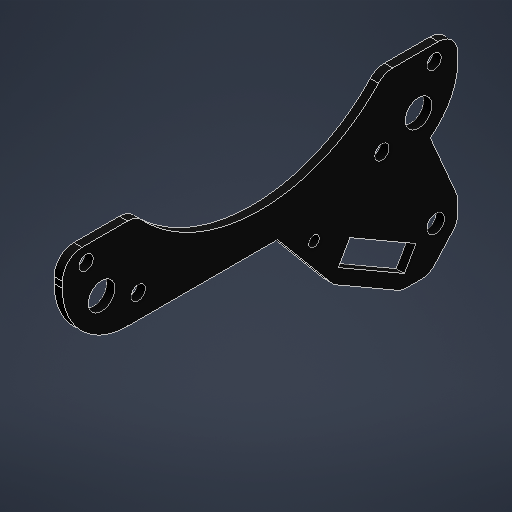
# Autodesk Inventor part: output_support
Saved by Autodesk Inventor 2026.1 (Build 301233000, 233)
## iProperties
Created: 2026-05-06
Part Number: output_support
Material: Generic
Document SubType Name: Modeling
Designer: aaron
Density: 1 g/cm^3
Appearance: Default
Author: aaron
Autodesk Inventor part; units mm, degrees
ref_plane "YZ Plane" through (0, 0, 0) normal (1, 0, 0) x (0, 1, 0)
ref_plane "XZ Plane" through (0, 0, 0) normal (0, 1, 0) x (-1, 0, 0)
sketch "Sketch1" plane through (0, 0, 0) normal (1, 0, 0) x (0, 1, 0)
  line L0 (14.231, -0.0045) -> (14.2475, -121.0044)
  circle A0 centre (46.8483, -60.5) radius 44 projected
  arc A1 (-10.6283, -58.8604) -> (-0.114, -93.6782) centre (46.8483, -60.5) ccw projected
  line L1 (-0.114, -93.6782) -> (2.9975, -94.9709) projected
  arc A2 (2.9975, -94.9709) -> (7.0992, -99.6298) centre (46.8483, -60.5) ccw projected
  line L2 (7.0992, -99.6298) -> (13.2859, -93.5395) projected
  arc A3 (-0.2275, -59.1156) -> (13.2859, -93.5395) centre (46.8483, -60.5) ccw projected
  line L3 (-0.2275, -59.1156) -> (-8.9052, -58.8604) projected
  line L4 (-8.9052, -58.8604) -> (-10.6283, -58.8604) projected
  circle A4 centre (84.1308, -7.2551) radius 2.15 projected
  circle A5 centre (95.3483, -109) radius 2.65 projected
  circle A6 centre (100.0932, -97.7825) radius 2.15 projected
  circle A7 centre (-6.3966, -23.2175) radius 2.15 projected
  circle A8 centre (-6.3966, -97.7825) radius 2.15 projected
  circle A9 centre (-1.6517, -12) radius 2.65 projected
  circle A10 centre (95.3483, -12) radius 2.65 projected
  circle A11 centre (9.5658, -113.7449) radius 2.15 projected
  circle A12 centre (9.5658, -7.2551) radius 2.15 projected
  circle A13 centre (84.1308, -113.7449) radius 2.15 projected
  circle A14 centre (100.0932, -23.2175) radius 2.15 projected
  circle A15 centre (-1.6517, -109) radius 2.65 projected
  line L5 (-7.7476, -49.0794) -> (0.7499, -50.8569) projected
  arc A16 (12.1591, -28.6456) -> (0.7499, -50.8569) centre (46.8483, -60.5) ccw projected
  line L6 (12.1591, -28.6456) -> (5.7646, -22.7737) projected
  arc A17 (5.7646, -22.7737) -> (-7.7476, -49.0794) centre (46.8483, -60.5) ccw projected
  line L7 (83.7453, -102.33) -> (78.0025, -95.8194) projected
  arc A18 (66.2911, -103.3955) -> (78.0025, -95.8194) centre (46.8483, -60.5) ccw projected
  line L8 (66.2911, -103.3955) -> (69.8751, -111.3026) projected
  arc A19 (69.8751, -111.3026) -> (83.7453, -102.33) centre (46.8483, -60.5) ccw projected
  line L9 (85.3896, -20.1799) -> (79.3909, -26.4555) projected
  arc A20 (89.1056, -39.7066) -> (79.3909, -26.4555) centre (46.8483, -60.5) ccw projected
  line L10 (89.1056, -39.7066) -> (96.8951, -35.8737) projected
  arc A21 (96.8951, -35.8737) -> (85.3896, -20.1799) centre (46.8483, -60.5) ccw projected
  line L11 (58.0786, -115.1353) -> (56.3307, -106.6317) projected
  arc A22 (42.4628, -107.3915) -> (56.3307, -106.6317) centre (46.8483, -60.5) ccw projected
  line L12 (42.4628, -107.3915) -> (41.6544, -116.0352) projected
  arc A23 (41.6544, -116.0352) -> (58.0786, -115.1353) centre (46.8483, -60.5) ccw projected
  line L13 (11.1274, -17.6613) -> (16.6872, -24.3288) projected
  arc A24 (31.0571, -16.1301) -> (16.6872, -24.3288) centre (46.8483, -60.5) ccw projected
  line L14 (31.0571, -16.1301) -> (28.1463, -7.9512) projected
  arc A25 (28.1463, -7.9512) -> (11.1274, -17.6613) centre (46.8483, -60.5) ccw projected
  line L15 (101.6271, -71.0083) -> (93.1011, -69.3728) projected
  arc A26 (82.2782, -91.5285) -> (93.1011, -69.3728) centre (46.8483, -60.5) ccw projected
  line L16 (82.2782, -91.5285) -> (88.8092, -97.2481) projected
  arc A27 (88.8092, -97.2481) -> (101.6271, -71.0083) centre (46.8483, -60.5) ccw projected
  line L17 (100.5451, -45.4072) -> (92.1875, -47.7563) projected
  arc A28 (93.8596, -63.3257) -> (92.1875, -47.7563) centre (46.8483, -60.5) ccw projected
  line L18 (93.8596, -63.3257) -> (102.5254, -63.8466) projected
  arc A29 (102.5254, -63.8466) -> (100.5451, -45.4072) centre (46.8483, -60.5) ccw projected
  line L19 (38.2646, -115.6131) -> (39.6006, -107.0351) projected
  arc A30 (20.5997, -99.6032) -> (39.6006, -107.0351) centre (46.8483, -60.5) ccw projected
  line L20 (20.5997, -99.6032) -> (15.7612, -106.8113) projected
  arc A31 (15.7612, -106.8113) -> (38.2646, -115.6131) centre (46.8483, -60.5) ccw projected
  line L21 (38.8508, -5.2987) -> (40.0955, -13.8905) projected
  arc A32 (56.4914, -14.4016) -> (40.0955, -13.8905) centre (46.8483, -60.5) ccw projected
  line L22 (56.4914, -14.4016) -> (58.2689, -5.9041) projected
  arc A33 (58.2689, -5.9041) -> (38.8508, -5.2987) centre (46.8483, -60.5) ccw projected
  arc A34 (6.34, -0.0055) -> (-13.6572, -20.0083) centre (6.3428, -20.0055) ccw projected
  line L23 (6.34, -0.0055) -> (87.34, 0.0055) projected
  arc A35 (107.3428, -19.9917) -> (87.34, 0.0055) centre (87.3428, -19.9945) ccw projected
  line L24 (107.3428, -19.9917) -> (107.3538, -100.9917) projected
  arc A36 (87.3566, -120.9945) -> (107.3538, -100.9917) centre (87.3538, -100.9945) ccw projected
  line L25 (87.3566, -120.9945) -> (6.3566, -121.0055) projected
  arc A37 (-13.6462, -101.0083) -> (6.3566, -121.0055) centre (6.3538, -101.0055) ccw projected
  line L26 (-13.6462, -101.0083) -> (-13.6572, -20.0083) projected
  line L27 (-13.651, -65.8198) -> (-34.151, -83.0261)
  line L28 (-34.151, -83.0261) -> (-46.1481, -103.8124)
  line L29 (-46.1481, -103.8124) -> (-46.1481, -112.3124)
  line L30 (-46.1481, -112.3124) -> (-36.5178, -121.0114)
  line L31 (-36.5178, -121.0114) -> (-13.6462, -101.0083)
  circle A38 centre (46.8483, -60.5) radius 50
  circle A39 centre (-1.6517, -109) radius 5.75 projected
  line L32 (-69.3325, -76.5758) -> (-2.1613, -115.3449)
  line L33 (-36.5178, -121.0114) -> (-29.7828, -121.0105)
  line L34 (-29.7828, -121.0105) -> (-1.6517, -109)
  point P0 (0, 0)
  point P1 (14.2445, -98.4076)
  point P2 (14.2341, -22.6013)
  point P3 (-9.9753, -112.5537)
  dimension "d4" = 100
  dimension "d5" = 60
  dimension "d6" = 90
  dimension "d7" = 12
  dimension "d8" = 12
  dimension "d26" = 8.5
  dimension "d27" = 20.5
  dimension "d29" = 0
  dimension "d36" = 50
  constraints: 18 end point, 3 point on line, 2 perpendicular, 1 centre point, 1 coincident, 1 collinear, 1 tangent, 1 vertical
  measures "d4" diameter of A38
  measures "d5" angle of L32 L0
  measures "d6" angle of L28 L32
  measures "d7" distance from line of L32 L27.end
  measures "d8" distance from line of L32 L28.end
  measures "d26" distance of L28.end L29.end
  measures "d27" horizontal distance of L27.start L27.end
  measures "d29" distance between parallel lines of L25 L33
  measures "d36" angle of L26 L27
extrude "Extrusion1" add sketch "Sketch1" along normal blind 2.54 contours L34 A39 L32 | L0 A25 L13 A38 L6 A17 L5 L3 L4 A1 L1 A2 L2 L25 A37 L34 L32 L26 A34 L23 | L0 L13 A25 | L26 L31 L32 L28 L27 | A38 L5 A17 L6 | A37 L32 L31 | L32 L34 A37 | A37 L34 L33 L31 L32 | L31 L30 L29 L28 L32 | A38 L2 A2 L1 A1 L4 L3 | A39
fillet "Fillet1" radius 6 4 edges at (1.27, 14.231, -0.0045) (1.27, 14.2475, -121.0044) (1.27, 14.2445, -98.4076) (1.27, 14.2341, -22.6013)
sketch "Sketch3" plane through (0, 0, 0) normal (-1, 0, 0) x (0, 0, 1)
  circle A0 centre (-12, -1.6517) radius 2.65 projected
  circle A1 centre (-12, -1.6517) radius 4.05
  circle A2 centre (-109, -1.6517) radius 2.65 projected
  circle A3 centre (-109, -1.6517) radius 4.05
  point P0 (0, 0)
  dimension "d13" = 8.1
  dimension "d14" = 8.1
  constraints: 2 centre point, 2 coincident
  measures "d13" diameter of A1
  measures "d14" diameter of A3
extrude "Extrusion3" cut sketch "Sketch3" against normal through all contours A0 | A1 | A2 | A3
ref_plane "Work Plane2" through (0, -42.6838, -105.8119) normal (0, -0.8661, 0.4999) x (1, 0, 0)
sketch "Sketch4" plane through (0, -42.6838, -105.8119) normal (0, -0.8661, 0.4999) x (1, 0, 0)
  circle A0 centre (-17.46, 13) radius 21
  line L0 (0, 24) -> (0, 0) projected
  line L1 (0, 24) -> (2.54, 24) projected
  line L2 (0, 49.1499) -> (0, 24) projected
  line L3 (0, 0) -> (0, -7.3618) projected
  line L4 (0, 1.3317) -> (3.4521, 1.3317)
  line L5 (3.4521, 1.3317) -> (7.9852, 19.2714)
  line L6 (0, 24.6683) -> (6.7025, 24.6683)
  line L7 (6.7025, 24.6683) -> (7.9852, 19.2714)
  line L8 (0, 13.7) -> (2.54, 13.7) projected
  line L9 (0, 11.3553) -> (2.54, 11.3553) projected
  line L10 (0, 11.3553) -> (0, 30.1698)
  point P0 (0, 112.9799)
  point P1 (0.4285, 24)
  point P2 (0, 24.6683)
  dimension "d18" = 42
  dimension "d19" = 17.46
  dimension "d30" = 0.7
  constraints: 10 end point, 3 point on line, 2 perpendicular, 2 point on circle, 1 centre point
  measures "d18" diameter of A0
  measures "d19" distance from line of A0.centre L0
  measures "d30" distance from line of A0.centre L8
extrude "Extrusion4" cut sketch "Sketch4" against normal blind 7.1 contours L6 L7 L5 L4 A0 | A0 L1 L2 | L0 L1 A0
sketch "Sketch5" plane through (0, 0, 0) normal (-1, 0, 0) x (0, 0, 1)
  circle A0 centre (-114.2363, -33.5753) radius 2.65
  line L0 (-112.3124, -46.1481) -> (-121.0114, -36.5178) projected
  line L1 (-108.2077, -35.8688) -> (-87.996, -24.2033) projected
  point P0 (0, 0)
  point P1 (-88.5749, -24.5372)
  dimension "d23" = 5.3
  dimension "d24" = 7
  dimension "d25" = 5
  constraints: 1 centre point, 1 other
  measures "d23" diameter of A0
  measures "d24" distance from line of L0 A0.centre
extrude "Extrusion5" cut sketch "Sketch5" against normal through all
sketch "Sketch6" plane through (0, 0, 0) normal (-1, 0, 0) x (0, 0, 1)
  circle A0 centre (-77, -19.6494) radius 1.6
  line L0 (-20.0083, -13.6572) -> (-65.8198, -13.651) projected
  circle A1 centre (-109, -1.6517) radius 4.05 projected
  point P0 (0, 0)
  dimension "d33" = 3.2
  dimension "d34" = 6
  dimension "d35" = 32
  constraints: 1 centre point
  measures "d33" diameter of A0
  measures "d34" distance from line of L0 A0.centre
  measures "d35" horizontal distance of A1.centre A0.centre
extrude "Extrusion6" cut sketch "Sketch6" against normal through all contours A0
fillet "Fillet2" radius 6 5 edges at (1.27, -34.151, -83.0261) (1.27, -46.1481, -103.8124) (1.27, -46.1481, -112.3124) (1.27, -36.5178, -121.0114) (1.27, -29.7828, -121.0105)
body "Solid1"
